Autodesk Inventor part; units mm, degrees
(part 6 of 6)
  spline S683 degree 3 poles (12.3188, -14.7027) (12.3363, -14.6737) (12.3539, -14.6449) (12.3717, -14.6162) knots 214 214 214 214 215 215 215 215
  line L2250 (12.3188, -14.7027) -> (12.3363, -14.6737) construction
  line L2251 (12.3363, -14.6737) -> (12.3539, -14.6449) construction
  line L2252 (12.3539, -14.6449) -> (12.3717, -14.6162) construction
  spline S684 degree 3 poles (12.3717, -14.6162) (12.3711, -14.659) (12.3735, -14.7022) (12.37, -14.7433) knots 215 215 215 215 216 216 216 216
  line L2253 (12.3717, -14.6162) -> (12.3711, -14.659) construction
  line L2254 (12.3711, -14.659) -> (12.3735, -14.7022) construction
  line L2255 (12.3735, -14.7022) -> (12.37, -14.7433) construction
  spline S685 degree 3 poles (12.37, -14.7433) (12.358, -14.8214) (12.334, -14.8994) (12.322, -14.9833) knots 216 216 216 216 217 217 217 217
  line L2256 (12.37, -14.7433) -> (12.358, -14.8214) construction
  line L2257 (12.358, -14.8214) -> (12.334, -14.8994) construction
  line L2258 (12.334, -14.8994) -> (12.322, -14.9833) construction
  spline S686 degree 3 poles (12.322, -14.9833) (12.31, -15.0613) (12.274, -15.1333) (12.262, -15.2113) knots 217 217 217 217 218 218 218 218
  line L2259 (12.322, -14.9833) -> (12.31, -15.0613) construction
  line L2260 (12.31, -15.0613) -> (12.274, -15.1333) construction
  line L2261 (12.274, -15.1333) -> (12.262, -15.2113) construction
  spline S687 degree 3 poles (12.262, -15.2113) (12.25, -15.2833) (12.226, -15.3373) (12.232, -15.4093) knots 218 218 218 218 219 219 219 219
  line L2262 (12.262, -15.2113) -> (12.25, -15.2833) construction
  line L2263 (12.25, -15.2833) -> (12.226, -15.3373) construction
  line L2264 (12.226, -15.3373) -> (12.232, -15.4093) construction
  spline S688 degree 3 poles (12.232, -15.4093) (12.232, -15.4513) (12.238, -15.4933) (12.244, -15.5293) knots 219 219 219 219 220 220 220 220
  line L2265 (12.232, -15.4093) -> (12.232, -15.4513) construction
  line L2266 (12.232, -15.4513) -> (12.238, -15.4933) construction
  line L2267 (12.238, -15.4933) -> (12.244, -15.5293) construction
  spline S689 degree 3 poles (12.244, -15.5293) (12.25, -15.5773) (12.28, -15.6073) (12.31, -15.6433) knots 220 220 220 220 221 221 221 221
  line L2268 (12.244, -15.5293) -> (12.25, -15.5773) construction
  line L2269 (12.25, -15.5773) -> (12.28, -15.6073) construction
  line L2270 (12.28, -15.6073) -> (12.31, -15.6433) construction
  spline S690 degree 3 poles (12.31, -15.6433) (12.412, -15.7633) (12.55, -15.8593) (12.706, -15.9013) knots 221 221 221 221 222 222 222 222
  line L2271 (12.31, -15.6433) -> (12.412, -15.7633) construction
  line L2272 (12.412, -15.7633) -> (12.55, -15.8593) construction
  line L2273 (12.55, -15.8593) -> (12.706, -15.9013) construction
  spline S691 degree 3 poles (12.706, -15.9013) (12.814, -15.9313) (12.91, -15.9253) (13.012, -15.8713) knots 222 222 222 222 223 223 223 223
  line L2274 (12.706, -15.9013) -> (12.814, -15.9313) construction
  line L2275 (12.814, -15.9313) -> (12.91, -15.9253) construction
  line L2276 (12.91, -15.9253) -> (13.012, -15.8713) construction
  spline S692 degree 3 poles (13.012, -15.8713) (13.156, -15.7933) (13.282, -15.6733) (13.39, -15.5593) knots 223 223 223 223 224 224 224 224
  line L2277 (13.012, -15.8713) -> (13.156, -15.7933) construction
  line L2278 (13.156, -15.7933) -> (13.282, -15.6733) construction
  line L2279 (13.282, -15.6733) -> (13.39, -15.5593) construction
  spline S693 degree 3 poles (13.39, -15.5593) (13.492, -15.4453) (13.57, -15.3193) (13.66, -15.1993) knots 224 224 224 224 225 225 225 225
  line L2280 (13.39, -15.5593) -> (13.492, -15.4453) construction
  line L2281 (13.492, -15.4453) -> (13.57, -15.3193) construction
  line L2282 (13.57, -15.3193) -> (13.66, -15.1993) construction
  spline S694 degree 3 poles (13.66, -15.1993) (13.744, -15.0913) (13.846, -14.9893) (13.93, -14.8813) knots 225 225 225 225 226 226 226 226
  line L2283 (13.66, -15.1993) -> (13.744, -15.0913) construction
  line L2284 (13.744, -15.0913) -> (13.846, -14.9893) construction
  line L2285 (13.846, -14.9893) -> (13.93, -14.8813) construction
  line L2286 (13.93, -14.8813) -> (14.254, -14.4614)
  line L2287 (14.254, -14.4614) -> (14.44, -14.2154)
  spline S695 degree 3 poles (14.44, -14.2154) (14.47, -14.1794) (14.4882, -14.1494) (14.4642, -14.1014) knots 228 228 228 228 229 229 229 229
  line L2288 (14.44, -14.2154) -> (14.47, -14.1794) construction
  line L2289 (14.47, -14.1794) -> (14.4882, -14.1494) construction
  line L2290 (14.4882, -14.1494) -> (14.4642, -14.1014) construction
  spline S696 degree 3 poles (14.4642, -14.1014) (14.4642, -14.1074) (14.4583, -14.1074) (14.4583, -14.1014) knots 229 229 229 229 230 230 230 230
  line L2291 (14.4642, -14.1014) -> (14.4642, -14.1074) construction
  line L2292 (14.4642, -14.1074) -> (14.4583, -14.1074) construction
  line L2293 (14.4583, -14.1074) -> (14.4583, -14.1014) construction
  line L2294 (9.472, -13.0754) -> (9.466, -13.0934)
  spline S697 degree 3 poles (9.466, -13.0934) (9.466, -13.0874) (9.466, -13.0814) (9.472, -13.0754) knots 1 1 1 1 2 2 2 2
  line L2295 (9.466, -13.0934) -> (9.466, -13.0874) construction
  line L2296 (9.466, -13.0874) -> (9.466, -13.0814) construction
  line L2297 (9.466, -13.0814) -> (9.472, -13.0754) construction
  spline S698 degree 3 poles (9.472, -13.0754) (9.472, -13.0694) (9.478, -13.0694) (9.478, -13.0694) knots 2 2 2 2 3 3 3 3
  line L2298 (9.472, -13.0754) -> (9.472, -13.0694) construction
  line L2299 (9.472, -13.0694) -> (9.478, -13.0694) construction
  line L2300 (9.478, -13.0694) -> (9.478, -13.0694) construction
  line L2301 (9.478, -13.0694) -> (9.472, -13.0754)
  spline S699 degree 3 poles (10.018, -11.9894) (9.988, -11.9834) (9.952, -12.0914) (9.904, -12.1994) (9.952, -12.0974) (10.012, -11.9894) (10.018, -11.9894) knots 0 0 0 0 1 1 1 2 2 2 2
  line L2302 (10.018, -11.9894) -> (9.988, -11.9834) construction
  line L2303 (9.988, -11.9834) -> (9.952, -12.0914) construction
  line L2304 (9.952, -12.0914) -> (9.904, -12.1994) construction
  line L2305 (9.904, -12.1994) -> (9.952, -12.0974) construction
  line L2306 (9.952, -12.0974) -> (10.012, -11.9894) construction
  line L2307 (10.012, -11.9894) -> (10.018, -11.9894) construction
  spline S700 degree 3 poles (9.472, -13.0754) (9.466, -13.0814) (9.466, -13.0874) (9.466, -13.0934) knots 0 0 0 0 1 1 1 1
  line L2308 (9.472, -13.0754) -> (9.466, -13.0814) construction
  line L2309 (9.466, -13.0814) -> (9.466, -13.0874) construction
  line L2310 (9.466, -13.0874) -> (9.466, -13.0934) construction
  line L2311 (9.466, -13.0934) -> (9.472, -13.0754)
  line L2312 (9.472, -13.0754) -> (9.478, -13.0694)
  spline S701 degree 3 poles (9.478, -13.0694) (9.478, -13.0694) (9.472, -13.0694) (9.472, -13.0754) knots 1 1 1 1 2 2 2 2
  line L2313 (9.478, -13.0694) -> (9.478, -13.0694) construction
  line L2314 (9.478, -13.0694) -> (9.472, -13.0694) construction
  line L2315 (9.472, -13.0694) -> (9.472, -13.0754) construction
  line L2316 (6.2561, -12.9614) -> (6.2321, -12.9974)
  spline S702 degree 3 poles (6.2321, -12.9974) (6.2321, -12.9974) (6.2441, -12.9854) (6.2561, -12.9614) knots 1 1 1 1 2 2 2 2
  line L2317 (6.2321, -12.9974) -> (6.2321, -12.9974) construction
  line L2318 (6.2321, -12.9974) -> (6.2441, -12.9854) construction
  line L2319 (6.2441, -12.9854) -> (6.2561, -12.9614) construction
  spline S703 degree 3 poles (5.4821, -14.7913) (5.3501, -14.7794) (5.2061, -14.7734) (5.0681, -14.7794) knots 0 0 0 0 1 1 1 1
  line L2320 (5.4821, -14.7913) -> (5.3501, -14.7794) construction
  line L2321 (5.3501, -14.7794) -> (5.2061, -14.7734) construction
  line L2322 (5.2061, -14.7734) -> (5.0681, -14.7794) construction
  spline S704 degree 3 poles (5.0681, -14.7794) (4.6541, -14.8033) (4.2401, -14.9054) (3.8441, -15.0253) knots 1 1 1 1 2 2 2 2
  line L2323 (5.0681, -14.7794) -> (4.6541, -14.8033) construction
  line L2324 (4.6541, -14.8033) -> (4.2401, -14.9054) construction
  line L2325 (4.2401, -14.9054) -> (3.8441, -15.0253) construction
  spline S705 degree 3 poles (3.8441, -15.0253) (4.1441, -14.2634) (4.2941, -13.4534) (4.5521, -12.6734) knots 2 2 2 2 3 3 3 3
  line L2326 (3.8441, -15.0253) -> (4.1441, -14.2634) construction
  line L2327 (4.1441, -14.2634) -> (4.2941, -13.4534) construction
  line L2328 (4.2941, -13.4534) -> (4.5521, -12.6734) construction
  spline S706 degree 3 poles (4.5521, -12.6734) (4.6781, -12.2954) (4.8161, -11.8754) (5.0621, -11.5574) knots 3 3 3 3 4 4 4 4
  line L2329 (4.5521, -12.6734) -> (4.6781, -12.2954) construction
  line L2330 (4.6781, -12.2954) -> (4.8161, -11.8754) construction
  line L2331 (4.8161, -11.8754) -> (5.0621, -11.5574) construction
  spline S707 degree 3 poles (5.0621, -11.5574) (5.1161, -11.4854) (5.2481, -11.3234) (5.3621, -11.3534) knots 4 4 4 4 5 5 5 5
  line L2332 (5.0621, -11.5574) -> (5.1161, -11.4854) construction
  line L2333 (5.1161, -11.4854) -> (5.2481, -11.3234) construction
  line L2334 (5.2481, -11.3234) -> (5.3621, -11.3534) construction
  spline S708 degree 3 poles (5.3621, -11.3534) (5.4581, -11.3834) (5.4101, -11.6294) (5.3921, -11.6954) knots 5 5 5 5 6 6 6 6
  line L2335 (5.3621, -11.3534) -> (5.4581, -11.3834) construction
  line L2336 (5.4581, -11.3834) -> (5.4101, -11.6294) construction
  line L2337 (5.4101, -11.6294) -> (5.3921, -11.6954) construction
  spline S709 degree 3 poles (5.3921, -11.6954) (5.4161, -11.6114) (5.5181, -11.2694) (5.2721, -11.3594) knots 6 6 6 6 7 7 7 7
  line L2338 (5.3921, -11.6954) -> (5.4161, -11.6114) construction
  line L2339 (5.4161, -11.6114) -> (5.5181, -11.2694) construction
  line L2340 (5.5181, -11.2694) -> (5.2721, -11.3594) construction
  spline S710 degree 3 poles (5.2721, -11.3594) (5.0081, -11.4554) (4.8521, -11.8394) (4.7501, -12.0734) knots 7 7 7 7 8 8 8 8
  line L2341 (5.2721, -11.3594) -> (5.0081, -11.4554) construction
  line L2342 (5.0081, -11.4554) -> (4.8521, -11.8394) construction
  line L2343 (4.8521, -11.8394) -> (4.7501, -12.0734) construction
  spline S711 degree 3 poles (4.7501, -12.0734) (4.8401, -11.8574) (4.9421, -11.6174) (5.1101, -11.4494) knots 8 8 8 8 9 9 9 9
  line L2344 (4.7501, -12.0734) -> (4.8401, -11.8574) construction
  line L2345 (4.8401, -11.8574) -> (4.9421, -11.6174) construction
  line L2346 (4.9421, -11.6174) -> (5.1101, -11.4494) construction
  spline S712 degree 3 poles (5.1101, -11.4494) (5.1821, -11.3834) (5.3561, -11.2514) (5.4341, -11.3654) knots 9 9 9 9 10 10 10 10
  line L2347 (5.1101, -11.4494) -> (5.1821, -11.3834) construction
  line L2348 (5.1821, -11.3834) -> (5.3561, -11.2514) construction
  line L2349 (5.3561, -11.2514) -> (5.4341, -11.3654) construction
  spline S713 degree 3 poles (5.4341, -11.3654) (5.5061, -11.4734) (5.4161, -11.7194) (5.3861, -11.8214) knots 10 10 10 10 11 11 11 11
  line L2350 (5.4341, -11.3654) -> (5.5061, -11.4734) construction
  line L2351 (5.5061, -11.4734) -> (5.4161, -11.7194) construction
  line L2352 (5.4161, -11.7194) -> (5.3861, -11.8214) construction
  spline S714 degree 3 poles (5.3861, -11.8214) (5.3261, -12.0194) (5.2481, -12.2174) (5.1581, -12.4034) knots 11 11 11 11 12 12 12 12
  line L2353 (5.3861, -11.8214) -> (5.3261, -12.0194) construction
  line L2354 (5.3261, -12.0194) -> (5.2481, -12.2174) construction
  line L2355 (5.2481, -12.2174) -> (5.1581, -12.4034) construction
  spline S715 degree 3 poles (5.1581, -12.4034) (5.1581, -12.3914) (5.2361, -12.1932) (5.2301, -12.1932) knots 12 12 12 12 13 13 13 13
  line L2356 (5.1581, -12.4034) -> (5.1581, -12.3914) construction
  line L2357 (5.1581, -12.3914) -> (5.2361, -12.1932) construction
  line L2358 (5.2361, -12.1932) -> (5.2301, -12.1932) construction
  spline S716 degree 3 poles (5.2301, -12.1932) (5.2061, -12.1872) (4.9963, -12.6246) (4.9961, -12.625) knots 13 13 13 13 14 14 14 14
  line L2359 (5.2301, -12.1932) -> (5.2061, -12.1872) construction
  line L2360 (5.2061, -12.1872) -> (4.9961, -12.625) construction
  line L2361 (4.9961, -12.625) -> (4.9961, -12.625) construction
  line L2362 (4.9961, -12.625) -> (5.0021, -12.625)
  spline S717 degree 3 poles (5.0021, -12.625) (4.9961, -12.6667) (4.9841, -12.6492) (4.9841, -12.6492) knots 15 15 15 15 16 16 16 16
  line L2363 (5.0021, -12.625) -> (4.9961, -12.6667) construction
  line L2364 (4.9961, -12.6667) -> (4.9841, -12.6492) construction
  line L2365 (4.9841, -12.6492) -> (4.9841, -12.6492) construction
  spline S718 degree 3 poles (4.9841, -12.6492) (4.9361, -12.7392) (5.0321, -12.7843) (5.1101, -12.7903) knots 16 16 16 16 17 17 17 17
  line L2366 (4.9841, -12.6492) -> (4.9361, -12.7392) construction
  line L2367 (4.9361, -12.7392) -> (5.0321, -12.7843) construction
  line L2368 (5.0321, -12.7843) -> (5.1101, -12.7903) construction
  spline S719 degree 3 poles (5.1101, -12.7903) (5.2301, -12.8023) (5.3621, -12.7438) (5.4581, -12.6718) knots 17 17 17 17 18 18 18 18
  line L2369 (5.1101, -12.7903) -> (5.2301, -12.8023) construction
  line L2370 (5.2301, -12.8023) -> (5.3621, -12.7438) construction
  line L2371 (5.3621, -12.7438) -> (5.4581, -12.6718) construction
  spline S720 degree 3 poles (5.4581, -12.6718) (5.7101, -12.4798) (5.9261, -12.0306) (5.9081, -11.7126) knots 18 18 18 18 19 19 19 19
  line L2372 (5.4581, -12.6718) -> (5.7101, -12.4798) construction
  line L2373 (5.7101, -12.4798) -> (5.9261, -12.0306) construction
  line L2374 (5.9261, -12.0306) -> (5.9081, -11.7126) construction
  spline S721 degree 3 poles (5.9081, -11.7126) (5.8901, -11.4546) (5.7941, -11.269) (5.5421, -11.131) knots 19 19 19 19 20 20 20 20
  line L2375 (5.9081, -11.7126) -> (5.8901, -11.4546) construction
  line L2376 (5.8901, -11.4546) -> (5.7941, -11.269) construction
  line L2377 (5.7941, -11.269) -> (5.5421, -11.131) construction
  spline S722 degree 3 poles (5.5421, -11.131) (5.4041, -11.053) (5.2301, -10.9932) (5.0621, -11.0052) knots 20 20 20 20 21 21 21 21
  line L2378 (5.5421, -11.131) -> (5.4041, -11.053) construction
  line L2379 (5.4041, -11.053) -> (5.2301, -10.9932) construction
  line L2380 (5.2301, -10.9932) -> (5.0621, -11.0052) construction
  spline S723 degree 3 poles (5.0621, -11.0052) (4.8221, -11.0172) (4.6361, -11.1733) (4.5041, -11.3653) knots 21 21 21 21 22 22 22 22
  line L2381 (5.0621, -11.0052) -> (4.8221, -11.0172) construction
  line L2382 (4.8221, -11.0172) -> (4.6361, -11.1733) construction
  line L2383 (4.6361, -11.1733) -> (4.5041, -11.3653) construction
  spline S724 degree 3 poles (4.5041, -11.3653) (4.4021, -11.5213) (4.3361, -11.6894) (4.2761, -11.8574) knots 22 22 22 22 23 23 23 23
  line L2384 (4.5041, -11.3653) -> (4.4021, -11.5213) construction
  line L2385 (4.4021, -11.5213) -> (4.3361, -11.6894) construction
  line L2386 (4.3361, -11.6894) -> (4.2761, -11.8574) construction
  line L2387 (4.2761, -11.8574) -> (4.1921, -12.1094)
  spline S725 degree 3 poles (4.1921, -12.1094) (4.1681, -12.1754) (4.1021, -12.2834) (4.1141, -12.3494) knots 24 24 24 24 25 25 25 25
  line L2388 (4.1921, -12.1094) -> (4.1681, -12.1754) construction
  line L2389 (4.1681, -12.1754) -> (4.1021, -12.2834) construction
  line L2390 (4.1021, -12.2834) -> (4.1141, -12.3494) construction
  spline S726 degree 3 poles (4.1141, -12.3494) (4.1141, -12.3614) (4.1561, -12.2714) (4.1621, -12.2654) knots 25 25 25 25 26 26 26 26
  line L2391 (4.1141, -12.3494) -> (4.1141, -12.3614) construction
  line L2392 (4.1141, -12.3614) -> (4.1561, -12.2714) construction
  line L2393 (4.1561, -12.2714) -> (4.1621, -12.2654) construction
  spline S727 degree 3 poles (4.1621, -12.2654) (4.1261, -12.3794) (4.0961, -12.4994) (4.0601, -12.6194) knots 26 26 26 26 27 27 27 27
  line L2394 (4.1621, -12.2654) -> (4.1261, -12.3794) construction
  line L2395 (4.1261, -12.3794) -> (4.0961, -12.4994) construction
  line L2396 (4.0961, -12.4994) -> (4.0601, -12.6194) construction
  spline S728 degree 3 poles (4.0601, -12.6194) (4.0541, -12.6134) (4.0781, -12.5294) (4.0721, -12.5294) (4.0421, -12.5294) (3.9401, -12.9134) (3.9281, -12.9434) knots 27 27 27 27 28 28 28 29 29 29 29
  line L2397 (4.0601, -12.6194) -> (4.0541, -12.6134) construction
  line L2398 (4.0541, -12.6134) -> (4.0781, -12.5294) construction
  line L2399 (4.0781, -12.5294) -> (4.0721, -12.5294) construction
  line L2400 (4.0721, -12.5294) -> (4.0421, -12.5294) construction
  line L2401 (4.0421, -12.5294) -> (3.9401, -12.9134) construction
  line L2402 (3.9401, -12.9134) -> (3.9281, -12.9434) construction
  spline S729 degree 3 poles (3.9281, -12.9434) (3.8681, -13.1594) (3.8021, -13.3814) (3.7781, -13.6094) knots 29 29 29 29 30 30 30 30
  line L2403 (3.9281, -12.9434) -> (3.8681, -13.1594) construction
  line L2404 (3.8681, -13.1594) -> (3.8021, -13.3814) construction
  line L2405 (3.8021, -13.3814) -> (3.7781, -13.6094) construction
  spline S730 degree 3 poles (3.7781, -13.6094) (3.7541, -13.8194) (3.7241, -14.0114) (3.6701, -14.2154) knots 30 30 30 30 31 31 31 31
  line L2406 (3.7781, -13.6094) -> (3.7541, -13.8194) construction
  line L2407 (3.7541, -13.8194) -> (3.7241, -14.0114) construction
  line L2408 (3.7241, -14.0114) -> (3.6701, -14.2154) construction
  spline S731 degree 3 poles (3.6701, -14.2154) (3.6461, -14.3294) (3.6101, -14.4374) (3.5801, -14.5514) knots 31 31 31 31 32 32 32 32
  line L2409 (3.6701, -14.2154) -> (3.6461, -14.3294) construction
  line L2410 (3.6461, -14.3294) -> (3.6101, -14.4374) construction
  line L2411 (3.6101, -14.4374) -> (3.5801, -14.5514) construction
  spline S732 degree 3 poles (3.5801, -14.5514) (3.5621, -14.6294) (3.4661, -14.8454) (3.4961, -14.9233) knots 32 32 32 32 33 33 33 33
  line L2412 (3.5801, -14.5514) -> (3.5621, -14.6294) construction
  line L2413 (3.5621, -14.6294) -> (3.4661, -14.8454) construction
  line L2414 (3.4661, -14.8454) -> (3.4961, -14.9233) construction
  spline S733 degree 3 poles (3.4961, -14.9233) (3.5021, -14.9293) (3.5081, -14.9293) (3.5141, -14.9233) knots 33 33 33 33 34 34 34 34
  line L2415 (3.4961, -14.9233) -> (3.5021, -14.9293) construction
  line L2416 (3.5021, -14.9293) -> (3.5081, -14.9293) construction
  line L2417 (3.5081, -14.9293) -> (3.5141, -14.9233) construction
  spline S734 degree 3 poles (3.5141, -14.9233) (3.4961, -14.9773) (3.4902, -15.0253) (3.4721, -15.0733) knots 34 34 34 34 35 35 35 35
  line L2418 (3.5141, -14.9233) -> (3.4961, -14.9773) construction
  line L2419 (3.4961, -14.9773) -> (3.4902, -15.0253) construction
  line L2420 (3.4902, -15.0253) -> (3.4721, -15.0733) construction
  spline S735 degree 3 poles (3.4721, -15.0733) (3.4722, -15.0732) (3.5021, -14.9473) (3.4961, -14.9473) knots 35 35 35 35 36 36 36 36
  line L2421 (3.4721, -15.0733) -> (3.4721, -15.0733) construction
  line L2422 (3.4721, -15.0733) -> (3.5021, -14.9473) construction
  line L2423 (3.5021, -14.9473) -> (3.4961, -14.9473) construction
  spline S736 degree 3 poles (3.4961, -14.9473) (3.4661, -14.9654) (3.4601, -15.1093) (3.4601, -15.1034) knots 36 36 36 36 37 37 37 37
  line L2424 (3.4961, -14.9473) -> (3.4661, -14.9654) construction
  line L2425 (3.4661, -14.9654) -> (3.4601, -15.1093) construction
  line L2426 (3.4601, -15.1093) -> (3.4601, -15.1034) construction
  spline S737 degree 3 poles (3.4601, -15.1034) (3.4242, -15.1993) (3.3101, -15.1993) (3.2202, -15.2413) knots 37 37 37 37 38 38 38 38
  line L2427 (3.4601, -15.1034) -> (3.4242, -15.1993) construction
  line L2428 (3.4242, -15.1993) -> (3.3101, -15.1993) construction
  line L2429 (3.3101, -15.1993) -> (3.2202, -15.2413) construction
  spline S738 degree 3 poles (3.2202, -15.2413) (3.1422, -15.2713) (3.0762, -15.3193) (3.0162, -15.3793) (2.8902, -15.5053) (2.7281, -15.7273) (2.7882, -15.9253) knots 38 38 38 38 39 39 39 40 40 40 40
  line L2430 (3.2202, -15.2413) -> (3.1422, -15.2713) construction
  line L2431 (3.1422, -15.2713) -> (3.0762, -15.3193) construction
  line L2432 (3.0762, -15.3193) -> (3.0162, -15.3793) construction
  line L2433 (3.0162, -15.3793) -> (2.8902, -15.5053) construction
  line L2434 (2.8902, -15.5053) -> (2.7281, -15.7273) construction
  line L2435 (2.7281, -15.7273) -> (2.7882, -15.9253) construction
  spline S739 degree 3 poles (2.7882, -15.9253) (2.8302, -16.0693) (2.9921, -16.1053) (3.1241, -16.0873) knots 40 40 40 40 41 41 41 41
  line L2436 (2.7882, -15.9253) -> (2.8302, -16.0693) construction
  line L2437 (2.8302, -16.0693) -> (2.9921, -16.1053) construction
  line L2438 (2.9921, -16.1053) -> (3.1241, -16.0873) construction
  spline S740 degree 3 poles (3.1241, -16.0873) (3.1841, -16.0753) (3.3701, -16.0153) (3.3582, -15.9373) knots 41 41 41 41 42 42 42 42
  line L2439 (3.1241, -16.0873) -> (3.1841, -16.0753) construction
  line L2440 (3.1841, -16.0753) -> (3.3701, -16.0153) construction
  line L2441 (3.3701, -16.0153) -> (3.3582, -15.9373) construction
  spline S741 degree 3 poles (3.3582, -15.9373) (3.3522, -15.9253) (3.2621, -15.9853) (3.2322, -15.9973) knots 42 42 42 42 43 43 43 43
  line L2442 (3.3582, -15.9373) -> (3.3522, -15.9253) construction
  line L2443 (3.3522, -15.9253) -> (3.2621, -15.9853) construction
  line L2444 (3.2621, -15.9853) -> (3.2322, -15.9973) construction
  line L2445 (3.2322, -15.9973) -> (3.2262, -16.0033)
  spline S742 degree 3 poles (3.2262, -16.0033) (3.2262, -16.0033) (3.2262, -15.9973) (3.2322, -15.9973) knots 44 44 44 44 45 45 45 45
  line L2446 (3.2262, -16.0033) -> (3.2262, -16.0033) construction
  line L2447 (3.2262, -16.0033) -> (3.2262, -15.9973) construction
  line L2448 (3.2262, -15.9973) -> (3.2322, -15.9973) construction
  spline S743 degree 3 poles (3.2322, -15.9973) (3.2741, -15.9673) (3.3221, -15.9253) (3.3582, -15.8893) knots 45 45 45 45 46 46 46 46
  line L2449 (3.2322, -15.9973) -> (3.2741, -15.9673) construction
  line L2450 (3.2741, -15.9673) -> (3.3221, -15.9253) construction
  line L2451 (3.3221, -15.9253) -> (3.3582, -15.8893) construction
  spline S744 degree 3 poles (3.3582, -15.8893) (3.3522, -15.9073) (3.4721, -15.7753) (3.4842, -15.7573) knots 46 46 46 46 47 47 47 47
  line L2452 (3.3582, -15.8893) -> (3.3522, -15.9073) construction
  line L2453 (3.3522, -15.9073) -> (3.4721, -15.7753) construction
  line L2454 (3.4721, -15.7753) -> (3.4842, -15.7573) construction
  spline S745 degree 3 poles (3.4842, -15.7573) (3.5502, -15.6673) (3.6281, -15.6313) (3.7241, -15.5833) knots 47 47 47 47 48 48 48 48
  line L2455 (3.4842, -15.7573) -> (3.5502, -15.6673) construction
  line L2456 (3.5502, -15.6673) -> (3.6281, -15.6313) construction
  line L2457 (3.6281, -15.6313) -> (3.7241, -15.5833) construction
  spline S746 degree 3 poles (3.7241, -15.5833) (3.8861, -15.4933) (4.0541, -15.4093) (4.2281, -15.3493) knots 48 48 48 48 49 49 49 49
  line L2458 (3.7241, -15.5833) -> (3.8861, -15.4933) construction
  line L2459 (3.8861, -15.4933) -> (4.0541, -15.4093) construction
  line L2460 (4.0541, -15.4093) -> (4.2281, -15.3493) construction
  spline S747 degree 3 poles (4.2281, -15.3493) (4.6001, -15.2173) (5.0081, -15.2053) (5.3621, -15.0253) knots 49 49 49 49 50 50 50 50
  line L2461 (4.2281, -15.3493) -> (4.6001, -15.2173) construction
  line L2462 (4.6001, -15.2173) -> (5.0081, -15.2053) construction
  line L2463 (5.0081, -15.2053) -> (5.3621, -15.0253) construction
  spline S748 degree 3 poles (5.3621, -15.0253) (5.4521, -14.9833) (5.6921, -14.8153) (5.4821, -14.7913) knots 50 50 50 50 51 51 51 51
  line L2464 (5.3621, -15.0253) -> (5.4521, -14.9833) construction
  line L2465 (5.4521, -14.9833) -> (5.6921, -14.8153) construction
  line L2466 (5.6921, -14.8153) -> (5.4821, -14.7913) construction
  point P0 (24.8539, -13.953)
sketch "Sketch2" plane through (0, 0, 0) normal (1, 0, 0) x (0, 1, 0)
  line L0 (0, 20) -> (0, -20)
  line L1 (0, -20) -> (30, -17.5)
  line L2 (30, -17.5) -> (30, 17.5)
  line L3 (30, 17.5) -> (0, 20)
  line L4 (0, 28) -> (0, -28) projected
  line L5 (0, -28) -> (0, 28) projected
  line L6 (-6, 0) -> (36, 0) projected
  point P0 (0, 0)
  dimension "d4" = 30
  dimension "d5" = 35
  dimension "d6" = 40
  constraints: 8 end point, 2 parallel, 1 collinear, 1 vertical, 1 other
  measures "d4" distance between parallel lines of L0 L2
  measures "d5" distance of L1.end L2.end
  measures "d6" distance of L0.start L0.end
extrude "Extrusion1" add sketch "Sketch2" against normal blind 2.5
sketch "Sketch5" plane through (0, 0, 0) normal (1, 0, 0) x (0, 0, -1)
  line L0 (-17.5, 30) -> (17.5, 30) projected
  line L1 (15, 30) -> (9.7102, 0)
  line L2 (9.7102, 0) -> (-9.6716, 0)
  line L3 (-9.6716, 0) -> (-16.9521, 41.2896)
  line L4 (-14.627, 42.5) -> (-7.5739, 2.5)
  line L5 (-7.5739, 2.5) -> (7.6124, 2.5)
  line L6 (7.6124, 2.5) -> (12.4614, 30)
  line L7 (12.4614, 30) -> (15, 30)
  line L8 (-20, 0) -> (20, 0) projected
  line L9 (-14.627, 42.5) -> (-24.627, 52.5)
  line L10 (-24.627, 52.5) -> (-26.3947, 50.7322)
  line L11 (-26.3947, 50.7322) -> (-16.9521, 41.2896)
  line L12 (0, -11.2653) -> (0, 67.592) projected
  point P0 (0, 0)
  dimension "d15" = 2.5
  dimension "d16" = 2.5
  dimension "d17" = 2.5
  dimension "d18" = 2.5
  dimension "d19" = 2.5
  dimension "d20" = 40
  dimension "d22" = 100
  dimension "d23" = 100
  dimension "d43" = 2.5
  dimension "d45" = 45
  dimension "d46" = 10
  constraints: 20 end point, 5 parallel, 1 collinear, 1 perpendicular, 1 point on line
  measures "d15" distance between parallel lines of L1 L6
  measures "d16" distance between parallel lines of L2 L5
  measures "d17" distance between parallel lines of L4 L3
  measures "d18" distance of L0.end L1.start
  measures "d19" distance from line of L3 L0.start
  measures "d20" vertical distance of L4.start L4.end
  measures "d22" angle of L5 L4
  measures "d23" angle of L5 L6
  measures "d43" distance of L9.end L10.end
  measures "d45" angle of L12 L9
  measures "d46" horizontal distance of L9.end L4.start
extrude "Extrusion2" add sketch "Sketch5" along normal blind 45 contours L0 L1 L2 L12 L5 L6 | L4 L5 L12 L2 L3 L0 | L0 L3 L11 L10 L9 L4
sketch "Sketch8" plane through (45, 30, -15) normal (0, -0.1736482, -0.9848078) x (-1, 0, 0)
  line L0 (0, 0) -> (25, 0)
  line L1 (25, 0) -> (25, -10)
  line L2 (25, -10) -> (0, -10)
  line L3 (0, -10) -> (0, 0)
  line L4 (45, 0) -> (0, 0) projected
  point P0 (45, -32.149)
  dimension "d33" = 10
  dimension "d34" = 25
  constraints: 8 end point, 2 parallel, 1 collinear, 1 horizontal, 1 perpendicular
  measures "d33" distance between parallel lines of L0 L2
  measures "d34" distance between parallel lines of L3 L1
extrude "Extrusion5" cut sketch "Sketch8" against normal blind 2.5
sketch "Sketch9" plane through (45, 42.5, 14.627) normal (0, 0.1736482, -0.9848078) x (-1, 0, 0)
  line L0 (45, 87.3072) -> (45, 60.7796)
  line L1 (45, 87.3072) -> (35, 87.3072)
  line L2 (35, 87.3072) -> (35, -12.6928)
  line L3 (35, -12.6928) -> (45, -12.6928)
  line L4 (45, -12.6928) -> (45, 87.3072)
  line L5 (45, -12.6928) -> (45, 0) projected
  point P0 (45, -44.3943)
  point P1 (45, -20)
  dimension "d38" = 10
  dimension "d47" = 100
  constraints: 10 end point, 2 parallel, 1 collinear, 1 horizontal, 1 perpendicular, 1 point on line
  measures "d38" distance of L2.end L3.end
  measures "d47" distance between parallel lines of L3 L1
extrude "Extrusion6" cut sketch "Sketch9" against normal through all
fillet "Fillet1" radius 2.5 6 edges at (10, 29.7829, 13.6539) (-1.25, 30, 17.5) (-1.25, 30, -17.5) (20, 30, -13.7307) (20, 20.369, -12.0325) (0, 29.7829, 13.6539)
mirror "Mirror1" about plane through (45, 26.25, 5.6974) normal (1, 0, 0)
equation "\"d15\" = thickness"
equation "\"d16\" = thickness"
equation "\"d17\" = thickness"
equation "\"d18\" = thickness"
equation "\"d19\" = thickness"
equation "\"d22\" = d23"
equation "\"d35\" = thickness"
equation "\"thickness\" = 2.5"
body "Solid1"
